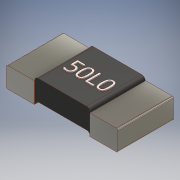
# Autodesk Inventor part: 21-0.05
Saved by Autodesk Inventor 2018 (Build 220112000, 112)
## iProperties
Created: 2019-09-21
Part Number: 21-0.05
Material: Copper
Document SubType Name: Modeling
Designer: Bradley
Density: 8.94 g/cm^3
Appearance: Copper - Satin
Author: Bradley
Autodesk Inventor part; units mm, degrees
ref_plane "YZ Plane" through (0, 0, 0) normal (1, 0, 0) x (0, 1, 0)
ref_plane "XZ Plane" through (0, 0, 0) normal (0, 1, 0) x (-1, 0, 0)
ref_plane "XY Plane" through (0, 0, 0) normal (0, 0, 1) x (1, 0, 0)
sketch "Sketch1" plane through (0, 0, 0) normal (0, 1, 0) x (-1, 0, 0)
  line L0 (0.379, 0.14) -> (-0.379, 0.14)
  line L1 (-0.379, 0.14) -> (-0.379, -0.14)
  line L2 (-0.379, -0.14) -> (0.379, -0.14)
  line L3 (0.379, -0.14) -> (0.379, 0.14)
  line L4 (0.379, 0.09) -> (0.76, 0.09)
  line L5 (0.76, 0.09) -> (0.76, -0.19)
  line L6 (0.76, -0.19) -> (0.379, -0.19)
  line L7 (0.379, -0.19) -> (0.379, 0.09)
  line L8 (-0.379, 0.09) -> (-0.76, 0.09)
  line L9 (-0.76, 0.09) -> (-0.76, -0.19)
  line L10 (-0.76, -0.19) -> (-0.379, -0.19)
  line L11 (-0.379, -0.19) -> (-0.379, 0.09)
  point P0 (0, 0)
  point P1 (0, 0.14)
  point P2 (0.379, 0)
  dimension "d0" = 0.381
  dimension "d1" = 1.52
  dimension "d2" = 0.05
  dimension "d3" = 0.33
  dimension "d4" = 0.05
  constraints: 24 end point, 6 parallel, 4 point on line, 3 horizontal, 3 perpendicular, 2 midpoint, 1 collinear, 1 horizontal alignment, 1 vertical alignment
  measures "d0" distance of L5.end L6.end
  measures "d1" distance between parallel lines of L5 L9
  measures "d2" distance between parallel lines of L6 L2
  measures "d3" distance between parallel lines of L6 L0
  measures "d4" distance between parallel lines of L0 L4
extrude "Extrusion1" add sketch "Sketch1" along normal mid plane 0.76 contours L4 L5 L6 L7 L3 | L1 L11 L10 L9 L8
extrude "Extrusion2" add sketch "Sketch1" along normal mid plane 0.75 contours L3 L2 L1 L0
fillet "Fillet1" radius 0.05 4 edges at (0.379, 0, 0.14) (-0.379, 0, 0.14) (-0.379, 0, -0.14) (0.379, 0, -0.14)
fillet "Fillet2" radius 0.02 4 edges at (-0.76, 0, 0.09) (-0.76, 0, -0.19) (0.76, 0, 0.09) (0.76, 0, -0.19)
sketch "Sketch2" plane through (-0.329, -0.375, 0.14) normal (0, 0, 1) x (1, 0, 0)
  line L0 (0, 0) -> (0, 0.75) projected
  line L1 (0.658, 0) -> (0, 0) projected
  line L2 (0.658, 0.75) -> (0.658, 0) projected
  line L3 (0, 0.75) -> (0.658, 0.75) construction
  line L4 (0, 0.375) -> (0.658, 0.375) construction
  spline S0 degree 2 poles (0.1713, 0.3385) (0.1713, 0.3241) (0.1621, 0.2995) (0.1536, 0.2904) knots 0 0 0 1 2 2 2
  spline S1 degree 2 poles (0.1536, 0.2904) (0.1452, 0.2813) (0.1201, 0.2708) (0.1045, 0.2708) knots 0 0 0 1 2 2 2
  spline S2 degree 2 poles (0.1045, 0.2708) (0.0903, 0.2708) (0.0624, 0.2771) (0.0522, 0.2821) knots 0 0 0 1 2 2 2
  line L5 (0.0522, 0.2821) -> (0.0522, 0.3105)
  line L6 (0.0522, 0.3105) -> (0.0541, 0.3105)
  spline S3 degree 2 poles (0.0541, 0.3105) (0.0572, 0.3082) (0.0687, 0.3024) (0.0757, 0.2998) knots 0 0 0 1 2 2 2
  spline S4 degree 2 poles (0.0757, 0.2998) (0.0836, 0.297) (0.0967, 0.294) (0.105, 0.294) knots 0 0 0 1 2 2 2
  spline S5 degree 2 poles (0.105, 0.294) (0.1131, 0.294) (0.1284, 0.2998) (0.1339, 0.3061) knots 0 0 0 1 2 2 2
  spline S6 degree 2 poles (0.1339, 0.3061) (0.1389, 0.3121) (0.1441, 0.328) (0.1441, 0.3387) knots 0 0 0 1 2 2 2
  spline S7 degree 2 poles (0.1441, 0.3387) (0.1441, 0.3494) (0.1382, 0.363) (0.1327, 0.3675) knots 0 0 0 1 2 2 2
  spline S8 degree 2 poles (0.1327, 0.3675) (0.1271, 0.3726) (0.1102, 0.3768) (0.1, 0.3768) knots 0 0 0 1 2 2 2
  spline S9 degree 2 poles (0.1, 0.3768) (0.089, 0.3768) (0.0671, 0.3734) (0.0604, 0.3719) knots 0 0 0 1 2 2 2
  line L7 (0.0604, 0.3719) -> (0.0604, 0.475)
  line L8 (0.0604, 0.475) -> (0.1702, 0.475)
  line L9 (0.1702, 0.475) -> (0.1702, 0.4515)
  line L10 (0.1702, 0.4515) -> (0.0862, 0.4515)
  line L11 (0.0862, 0.4515) -> (0.0862, 0.3982)
  spline S10 degree 2 poles (0.0862, 0.3982) (0.0911, 0.3988) (0.1005, 0.3993) (0.1044, 0.3993) knots 0 0 0 1 2 2 2
  spline S11 degree 2 poles (0.1044, 0.3993) (0.1198, 0.3993) (0.141, 0.3943) (0.1507, 0.3868) knots 0 0 0 1 2 2 2
  spline S12 degree 2 poles (0.1507, 0.3868) (0.1606, 0.3794) (0.1713, 0.3567) (0.1713, 0.3385) knots 0 0 0 1 2 2 2
  spline S13 degree 2 poles (0.3246, 0.375) (0.3246, 0.3212) (0.2933, 0.2708) (0.2608, 0.2708) knots 0 0 0 1 2 2 2
  spline S14 degree 2 poles (0.2608, 0.2708) (0.2277, 0.2708) (0.1967, 0.3222) (0.1967, 0.3748) knots 0 0 0 1 2 2 2
  spline S15 degree 2 poles (0.1967, 0.3748) (0.1967, 0.429) (0.228, 0.4791) (0.2608, 0.4791) knots 0 0 0 1 2 2 2
  spline S16 degree 2 poles (0.2608, 0.4791) (0.2937, 0.4791) (0.3246, 0.4272) (0.3246, 0.375) knots 0 0 0 1 2 2 2
  spline S17 degree 2 poles (0.2903, 0.3141) (0.2942, 0.3239) (0.2974, 0.3544) (0.2974, 0.375) knots 0 0 0 1 2 2 2
  spline S18 degree 2 poles (0.2974, 0.375) (0.2974, 0.3956) (0.2942, 0.4259) (0.2901, 0.4361) knots 0 0 0 1 2 2 2
  spline S19 degree 2 poles (0.2901, 0.4361) (0.2861, 0.4463) (0.2719, 0.4568) (0.2608, 0.4568) knots 0 0 0 1 2 2 2
  spline S20 degree 2 poles (0.2608, 0.4568) (0.2496, 0.4568) (0.2352, 0.4463) (0.2309, 0.4358) knots 0 0 0 1 2 2 2
  spline S21 degree 2 poles (0.2309, 0.4358) (0.2269, 0.4256) (0.224, 0.3944) (0.224, 0.3748) knots 0 0 0 1 2 2 2
  spline S22 degree 2 poles (0.224, 0.3748) (0.224, 0.3538) (0.2266, 0.3256) (0.2308, 0.3145) knots 0 0 0 1 2 2 2
  spline S23 degree 2 poles (0.2308, 0.3145) (0.2347, 0.3042) (0.2491, 0.293) (0.2608, 0.293) knots 0 0 0 1 2 2 2
  spline S24 degree 2 poles (0.2608, 0.293) (0.2718, 0.293) (0.2862, 0.3035) (0.2903, 0.3141) knots 0 0 0 1 2 2 2
  line L12 (0.4718, 0.275) -> (0.3559, 0.275)
  line L13 (0.3559, 0.275) -> (0.3559, 0.475)
  line L14 (0.3559, 0.475) -> (0.3825, 0.475)
  line L15 (0.3825, 0.475) -> (0.3825, 0.2987)
  line L16 (0.3825, 0.2987) -> (0.4718, 0.2987)
  line L17 (0.4718, 0.2987) -> (0.4718, 0.275)
  spline S25 degree 2 poles (0.6115, 0.375) (0.6115, 0.3212) (0.5802, 0.2708) (0.5476, 0.2708) knots 0 0 0 1 2 2 2
  spline S26 degree 2 poles (0.5476, 0.2708) (0.5146, 0.2708) (0.4836, 0.3222) (0.4836, 0.3748) knots 0 0 0 1 2 2 2
  spline S27 degree 2 poles (0.4836, 0.3748) (0.4836, 0.429) (0.5149, 0.4791) (0.5476, 0.4791) knots 0 0 0 1 2 2 2
  spline S28 degree 2 poles (0.5476, 0.4791) (0.5805, 0.4791) (0.6115, 0.4272) (0.6115, 0.375) knots 0 0 0 1 2 2 2
  spline S29 degree 2 poles (0.5771, 0.3141) (0.581, 0.3239) (0.5843, 0.3544) (0.5843, 0.375) knots 0 0 0 1 2 2 2
  spline S30 degree 2 poles (0.5843, 0.375) (0.5843, 0.3956) (0.581, 0.4259) (0.577, 0.4361) knots 0 0 0 1 2 2 2
  spline S31 degree 2 poles (0.577, 0.4361) (0.5729, 0.4463) (0.5588, 0.4568) (0.5476, 0.4568) knots 0 0 0 1 2 2 2
  spline S32 degree 2 poles (0.5476, 0.4568) (0.5365, 0.4568) (0.522, 0.4463) (0.5178, 0.4358) knots 0 0 0 1 2 2 2
  spline S33 degree 2 poles (0.5178, 0.4358) (0.5138, 0.4256) (0.5108, 0.3944) (0.5108, 0.3748) knots 0 0 0 1 2 2 2
  spline S34 degree 2 poles (0.5108, 0.3748) (0.5108, 0.3538) (0.5134, 0.3256) (0.5177, 0.3145) knots 0 0 0 1 2 2 2
  spline S35 degree 2 poles (0.5177, 0.3145) (0.5215, 0.3042) (0.536, 0.293) (0.5476, 0.293) knots 0 0 0 1 2 2 2
  spline S36 degree 2 poles (0.5476, 0.293) (0.5587, 0.293) (0.5731, 0.3035) (0.5771, 0.3141) knots 0 0 0 1 2 2 2
  point P0 (0.329, 0.375)
  constraints: 2 end point, 2 midpoint, 1 horizontal
extrude "Extrusion3" add sketch "Sketch2" along normal blind 0.01
body "Solid1"
